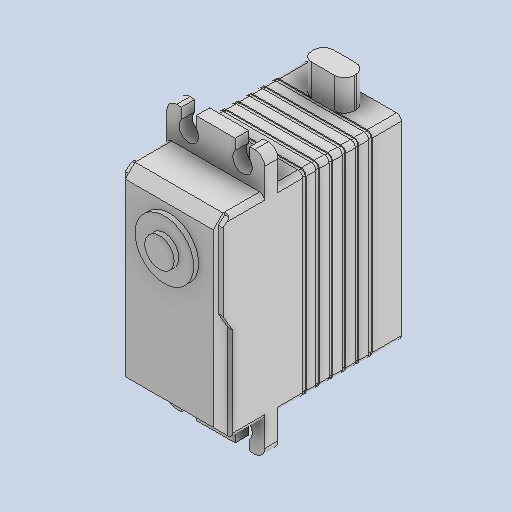
# Autodesk Inventor part: PerfectPass56KG
Saved by Autodesk Inventor 2025.2 (Build 292293000, 293)
## iProperties
Created: 2025-02-08
Part Number: PerfectPass56KG
Material: Generic
Document SubType Name: Modeling
Designer: LattePanda
Density: 1 g/cm^3
Appearance: Default
Author: LattePanda
Autodesk Inventor part; units mm, degrees
sketch "Sketch1" plane through (0, 0, 0) normal (0, 0, 1) x (1, 0, 0)
  line L0 (-10, -20) -> (10, -20)
  line L1 (10, -20) -> (10, 20)
  line L2 (10, 20) -> (-10, 20)
  line L3 (-10, 20) -> (-10, -20)
  line L4 (-10, -20) -> (10, 20) construction
  line L5 (10, -20) -> (-10, 20) construction
  point P0 (0, 0)
  dimension "d0" = 20
  dimension "d1" = 40
  constraints: 12 end point, 2 midpoint, 2 parallel, 1 horizontal, 1 perpendicular
  measures "d0" distance of L1.end L2.end
  measures "d1" distance of L0.end L1.end
extrude "Extrusion1" add sketch "Sketch1" against normal blind 37.5
fillet "Fillet1" radius 1 4 edges at (10, 20, -18.75) (10, -20, -18.75) (-10, -20, -18.75) (-10, 20, -18.75)
ref_plane "Work Plane1" through (0, 0, -9.5) normal (0, 0, 1) x (1, 0, 0)
sketch "Sketch2" plane through (0, 0, -9.5) normal (0, 0, 1) x (1, 0, 0)
  line L0 (-10, 27) -> (10, 27)
  line L1 (10, 27) -> (10, -27)
  line L2 (10, -27) -> (-10, -27)
  line L3 (-10, -27) -> (-10, 27)
  line L4 (-10, 19) -> (-10, -19) projected
  line L5 (10, -19) -> (10, 19) projected
  line L6 (9, 20) -> (-9, 20) projected
  line L7 (-9, -20) -> (9, -20) projected
  point P0 (0, 0)
  dimension "d6" = 54
  dimension "d7" = 7
  dimension "d8" = 7
  constraints: 8 end point, 2 collinear, 2 parallel, 1 horizontal, 1 perpendicular
  measures "d6" distance between parallel lines of L2 L0
  measures "d7" distance between parallel lines of L0 L6
  measures "d8" distance between parallel lines of L7 L2
extrude "Extrusion2" add sketch "Sketch2" against normal blind 2.75
fillet "Fillet2" radius 2 4 edges at (10, 27, -10.875) (-10, 27, -10.875) (10, -27, -10.875) (-10, -27, -10.875)
sketch "Sketch3" plane through (0, 0, -9.5) normal (0, 0, 1) x (1, 0, 0)
  circle A0 centre (-5.5, 23.482) radius 2
  line L0 (-8, 27) -> (8, 27) projected
  line L1 (0, 27) -> (0, -27) construction
  line L2 (-8, -27) -> (8, -27) projected
  line L3 (-7.5, 25.482) -> (-3.5, 25.482) construction
  line L4 (-3.5, 25.482) -> (-3.5, 21.482) construction
  line L5 (-3.5, 21.482) -> (-7.5, 21.482) construction
  line L6 (-7.5, 21.482) -> (-7.5, 25.482) construction
  line L7 (-10, 25) -> (-10, 19) projected
  circle A1 centre (5.5, 23.482) radius 2
  line L8 (-10, 19) -> (-10, -19) projected
  line L9 (10, -19) -> (10, 19) projected
  line L10 (-10, 0) -> (10, 0) construction
  circle A2 centre (-5.5, -23.482) radius 2
  circle A3 centre (5.5, -23.482) radius 2
  line L11 (-7, 24.8049) -> (-4, 24.8049)
  line L12 (-4, 24.8049) -> (-4, 27)
  line L13 (-4, 27) -> (-7, 27)
  line L14 (-7, 27) -> (-7, 24.8049)
  line L15 (4, 24.8049) -> (7, 24.8049)
  line L16 (7, 24.8049) -> (7, 27)
  line L17 (7, 27) -> (4, 27)
  line L18 (4, 27) -> (4, 24.8049)
  line L19 (-7, -24.8049) -> (-4, -24.8049)
  line L20 (-4, -24.8049) -> (-4, -27)
  line L21 (-7, -27) -> (-7, -24.8049)
  line L22 (4, -24.8049) -> (7, -24.8049)
  line L23 (7, -24.8049) -> (7, -27)
  line L24 (4, -27) -> (4, -24.8049)
  point P0 (0, 0)
  dimension "d12" = 4
  dimension "d13" = 2.5
  dimension "d14" = 3
  dimension "d15" = 3
  constraints: 40 end point, 11 symmetric about line, 6 parallel, 4 centre point, 4 midpoint, 4 point on circle, 4 tangent, 3 horizontal, 3 perpendicular, 2 point on line, 3 other
  measures "d12" diameter of A0
  measures "d13" distance between parallel lines of L7 L6
  measures "d14" distance between parallel lines of L12 L14
  measures "d15" distance of L15.start L15.end
extrude "Extrusion3" cut sketch "Sketch3" against normal blind 2.75
sketch "Sketch4" plane through (0, 0, 0) normal (0, 0, 1) x (1, 0, 0)
  line L0 (9, 20) -> (-9, 20) projected
  line L1 (0, 20) -> (0, 0)
  circle A0 centre (0, 10.5) radius 6
  dimension "d18" = 12
  dimension "d19" = 9.5
  constraints: 2 end point, 1 centre point, 1 midpoint, 1 point on line, 1 vertical
  measures "d18" diameter of A0
  measures "d19" distance from line of A0.centre L0
extrude "Extrusion4" add sketch "Sketch4" along normal blind 1
sketch "Sketch5" plane through (0, 10.5, 1) normal (0, 0, 1) x (1, 0, 0)
  circle A0 centre (0, 0) radius 6 projected
  circle A1 centre (0, 0) radius 3
  point P0 (0, -10.5)
  dimension "d22" = 6
  constraints: 1 centre point, 1 coincident
  measures "d22" diameter of A1
extrude "Extrusion5" add sketch "Sketch5" along normal blind 1 contours A1
ref_plane "Work Plane2" through (0, 0, -31.5) normal (0, 0, -1) x (-1, 0, 0)
sketch "Sketch6" plane through (0, 0, -31.5) normal (0, 0, -1) x (-1, 0, 0)
  arc A0 (10, 19) -> (9, 20) centre (9, 19) ccw projected
  line L0 (9, 20) -> (-9, 20) projected
  arc A1 (-9, 20) -> (-10, 19) centre (-9, 19) ccw projected
  line L1 (-10, 19) -> (-10, -19) projected
  arc A2 (-10, -19) -> (-9, -20) centre (-9, -19) ccw projected
  line L2 (-9, -20) -> (9, -20) projected
  arc A3 (9, -20) -> (10, -19) centre (9, -19) ccw projected
  line L3 (10, -19) -> (10, 19) projected
  line L4 (-9.8, -19) -> (-9.8, 19)
  arc A4 (-9, 19.8) -> (-9.8, 19) centre (-9, 19) ccw
  line L5 (-9, 19.8) -> (9, 19.8)
  arc A5 (9.8, 19) -> (9, 19.8) centre (9, 19) ccw
  line L6 (9.8, 19) -> (9.8, -19)
  arc A6 (9, -19.8) -> (9.8, -19) centre (9, -19) ccw
  line L7 (9, -19.8) -> (-9, -19.8)
  arc A7 (-9.8, -19) -> (-9, -19.8) centre (-9, -19) ccw
  point P0 (0, 0)
  dimension "d26" = 0.2
  constraints: 8 end point, 8 point on circle, 4 centre point, 7 other
  measures "d26" distance between parallel lines of L1 L4
extrude "Extrusion6" cut sketch "Sketch6" against normal blind 0.7
ref_plane "Work Plane3" through (0, 0, -28.8) normal (0, 0, -1) x (-1, 0, 0)
sketch "Sketch7" plane through (0, 0, -28.8) normal (0, 0, -1) x (-1, 0, 0)
  arc A0 (10, 19) -> (9, 20) centre (9, 19) ccw projected
  line L0 (9, 20) -> (-9, 20) projected
  arc A1 (-9, 20) -> (-10, 19) centre (-9, 19) ccw projected
  line L1 (-10, 19) -> (-10, -19) projected
  arc A2 (-10, -19) -> (-9, -20) centre (-9, -19) ccw projected
  line L2 (-9, -20) -> (9, -20) projected
  arc A3 (9, -20) -> (10, -19) centre (9, -19) ccw projected
  line L3 (10, -19) -> (10, 19) projected
  arc A4 (9.8, 19) -> (9, 19.8) centre (9, 19) ccw
  line L4 (9, 19.8) -> (-9, 19.8)
  arc A5 (-9, 19.8) -> (-9.8, 19) centre (-9, 19) ccw
  line L5 (-9.8, 19) -> (-9.8, -19)
  arc A6 (-9.8, -19) -> (-9, -19.8) centre (-9, -19) ccw
  line L6 (-9, -19.8) -> (9, -19.8)
  arc A7 (9, -19.8) -> (9.8, -19) centre (9, -19) ccw
  line L7 (9.8, -19) -> (9.8, 19)
  point P0 (0, 0)
  dimension "d30" = 0.2
  constraints: 8 end point, 8 point on circle, 4 centre point, 7 other
  measures "d30" distance between parallel lines of L3 L7
extrude "Extrusion7" cut sketch "Sketch7" against normal blind 0.7
sketch "Sketch8" plane through (-10, -19, 0) normal (-1, 0, 0) x (0, 0, 1)
  line L0 (-1, 37.3493) -> (-1, 21.6659)
  line L1 (-1, 21.6659) -> (-3, 18.2018)
  line L2 (-3, 18.2018) -> (-3, -1)
  line L3 (-1, 37.3493) -> (-2.3713, 38.5)
  line L4 (-2.3713, 38.5) -> (-2.3713, 39)
  line L5 (-9.5, 38) -> (0, 38) projected
  line L6 (0, 38) -> (0, 0) projected
  line L7 (-9.5, -1) -> (0, -1) projected
  line L8 (0, 39) -> (-9.5, 39) projected
  line L9 (0, 0) -> (0, -1) projected
  line L10 (0, 39) -> (0, 38) projected
  point P0 (0, 19)
  dimension "d33" = 1
  dimension "d34" = 3
  dimension "d35" = 0.5
  dimension "d36" = 40
  dimension "d37" = 150
  constraints: 10 end point, 2 parallel, 2 point on line, 1 perpendicular
  measures "d33" distance between parallel lines of L0 L6
  measures "d34" distance between parallel lines of L6 L2
  measures "d35" distance of L3.end L4.end
  measures "d36" angle of L8 L3
  measures "d37" angle of L2 L1
extrude "Extrusion8" cut sketch "Sketch8" against normal blind 1
mirror "Mirror1" about plane through (0, 0, 0) normal (1, 0, 0) of "Extrusion8"
chamfer "Chamfer1" distance 2 angle 45 1 edges at (0, 20, 0)
chamfer "Chamfer2" distance 3 angle 45 1 edges at (0, -20, 0)
ref_plane "Work Plane4" through (0, 0, -26.1) normal (0, 0, -1) x (-1, 0, 0)
sketch "Sketch9" plane through (0, 0, -26.1) normal (0, 0, -1) x (-1, 0, 0)
  arc A0 (10, 19) -> (9, 20) centre (9, 19) ccw projected
  line L0 (9, 20) -> (-9, 20) projected
  arc A1 (-9, 20) -> (-10, 19) centre (-9, 19) ccw projected
  line L1 (-10, 19) -> (-10, -19) projected
  arc A2 (-10, -19) -> (-9, -20) centre (-9, -19) ccw projected
  line L2 (-9, -20) -> (9, -20) projected
  arc A3 (9, -20) -> (10, -19) centre (9, -19) ccw projected
  line L3 (10, -19) -> (10, 19) projected
  arc A4 (9.8, 19) -> (9, 19.8) centre (9, 19) ccw
  line L4 (9.8, 19) -> (9.8, -19)
  arc A5 (9, -19.8) -> (9.8, -19) centre (9, -19) ccw
  line L5 (9, -19.8) -> (-9, -19.8)
  arc A6 (-9.8, -19) -> (-9, -19.8) centre (-9, -19) ccw
  line L6 (-9.8, -19) -> (-9.8, 19)
  arc A7 (-9, 19.8) -> (-9.8, 19) centre (-9, 19) ccw
  line L7 (-9, 19.8) -> (9, 19.8)
  point P0 (0, 0)
  dimension "d47" = 0.2
  constraints: 8 end point, 8 point on circle, 4 centre point, 7 other
  measures "d47" radial gap between concentric circles of A0 A4
extrude "Extrusion9" cut sketch "Sketch9" against normal blind 0.7
ref_plane "Work Plane5" through (0, 0, -24.4) normal (0, 0, -1) x (-1, 0, 0)
mirror "Mirror2" about plane through (0, 0, -24.4) normal (0, 0, -1) of "Extrusion9", "Extrusion7", "Extrusion6"
sketch "Sketch10" plane through (-9, 20, -37.5) normal (0, 1, 0) x (1, 0, 0)
  line L0 (0, -6) -> (18, -6) projected
  line L1 (18, 0) -> (18, -6) projected
  line L2 (0, 0) -> (18, 0) projected
  line L3 (0, -6) -> (0, 0) projected
  line L4 (9, 0) -> (9, -6) construction
  line L5 (13.325, -6) -> (4.675, -6)
  line L6 (4.675, -6) -> (4.675, -1.6)
  line L7 (4.675, -1.6) -> (13.325, -1.6)
  line L8 (13.325, -1.6) -> (13.325, -6)
  line L9 (13.325, -6) -> (4.675, -1.6) construction
  line L10 (4.675, -6) -> (13.325, -1.6) construction
  point P0 (9, -37.5)
  point P1 (9, -3.8)
  point P2 (4.675, -6)
  point P3 (13.325, -6)
  dimension "d51" = 8.65
  dimension "d52" = 4.4
  constraints: 14 end point, 4 midpoint, 2 parallel, 1 collinear, 1 horizontal, 1 perpendicular, 1 point on line
  measures "d51" distance of L6.end L7.end
  measures "d52" distance of L5.end L6.end
extrude "Extrusion10" add sketch "Sketch10" along normal blind 6.3 contours L6 L7 L8 L0
fillet "Fillet3" radius 2 4 edges at (-4.325, 23.15, -35.9) (4.325, 23.15, -35.9) (4.325, 23.15, -31.5) (-4.325, 23.15, -31.5)
equation "\"d8\" = d7"
body "Solid1"
